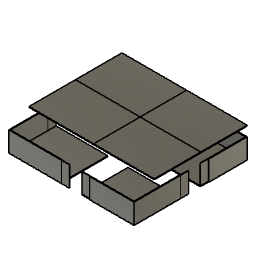
cajav3 v2 (Autodesk Fusion 360 design; units mm, degrees)
Autodesk Fusion 360 part; units mm, degrees
note: some values were not read from the file. Chosen so that the rebuilt part matches the saved one: which bodies a step acts on; which face or edge a step refers to.
sketch "Boceto1" plane through (0, 0, 0) normal (0, 0, 1) x (1, 0, 0)
  line L0 (0, 0) -> (-260, 0)
  line L1 (-260, 0) -> (-260, 230)
  line L2 (-260, 230) -> (0, 230)
  line L3 (0, 230) -> (0, 0)
  dimension "d1" = 230
  constraint horizontal L0
  constraint vertical L1
  constraint horizontal L2
  constraint vertical L3
  constraint coincident L0.start L3.end
  measures "d1" distance of L0.start L2.end
extrude "Extruir1" add sketch "Boceto1" along normal blind 50 and the other way blind 0 makes body 1
shell "Vaciado1" thickness 2 removed faces 1 at (-86.6667, 76.6667, 50) on bodies 1
ref_plane "PlanoDeObra1" through (-130, 0, 0) normal (1, 0, 0) x (0, 1, 0)
split "Dividir1" by plane through (-130, 0, 0) normal (1, 0, 0) bodies 1 makes body 2 at (-43.3333, 153.3333, 0)
move_body "Desplazar1" bodies 2 to x (1, 0, 0) y (0, 1, 0) z (0, 0, 1) at (50, 0, 0)
sketch "Boceto2" plane through (0, 0, 50) normal (0, 0, 1) x (-1, 0, 0)
  line L0 (80, -2) -> (80, 0)
  line L1 (80, 0) -> (-50, 0)
  line L2 (-50, 0) -> (-50, -230)
  line L3 (-50, -230) -> (80, -230)
  line L4 (80, -230) -> (80, -228)
  line L5 (80, -228) -> (-48, -228)
  line L6 (-48, -228) -> (-48, -2)
  line L7 (-48, -2) -> (80, -2)
  line L8 (80, 0) -> (60, 0)
  line L9 (60, 0) -> (60, -1)
  line L10 (60, -1) -> (80, -1)
  line L11 (80, -1) -> (80, 0)
  constraint horizontal L8
  constraint vertical L9
  constraint horizontal L10
  constraint vertical L11
  constraint coincident L0.end L1.start
extrude "Extruir2" cut sketch "Boceto2" against normal blind 51 contours L0 L1 L8 L9 L10 L11 bodies 2
sketch "Boceto3" plane through (-130, 0, 0) normal (1, 0, 0) x (0, 1, 0)
  line L0 (230, 0) -> (230, 50)
  line L1 (230, 50) -> (228, 50)
  line L2 (228, 50) -> (228, 2)
  line L3 (228, 2) -> (2, 2)
  line L4 (2, 2) -> (2, 50)
  line L5 (2, 50) -> (0, 50)
  line L6 (0, 50) -> (0, 0)
  line L7 (0, 0) -> (230, 0)
  line L8 (0, 0) -> (1, 0)
  line L9 (1, 0) -> (1, 50)
  line L10 (1, 50) -> (0, 50)
  line L11 (0, 50) -> (0, 0)
  dimension "d10" = 1
  constraint horizontal L8
  constraint vertical L9
  constraint horizontal L10
  constraint vertical L11
  constraint coincident L5 L9.end
  constraint coincident L6.end L7.start
  measures "d10" distance of L6.end L8.end
extrude "Extruir3" add sketch "Boceto3" along normal blind 20 and the other way blind 0 contours L5 L6 L7 L8 L9 L10 L11 bodies 1
sketch "Boceto4" plane through (-80, 0, 0) normal (-1, 0, 0) x (0, -1, 0)
  line L0 (-1, 0) -> (-1, 50)
  line L1 (-1, 50) -> (-2, 50)
  line L2 (-2, 50) -> (-2, 2)
  line L3 (-2, 2) -> (-228, 2)
  line L4 (-228, 2) -> (-228, 50)
  line L5 (-228, 50) -> (-230, 50)
  line L6 (-230, 50) -> (-230, 0)
  line L7 (-230, 0) -> (-1, 0)
  line L8 (-230, 0) -> (-229, 0)
  line L9 (-229, 0) -> (-229, 50)
  line L10 (-229, 50) -> (-230, 50)
  line L11 (-230, 50) -> (-230, 0)
  dimension "d15" = 1
  constraint horizontal L8
  constraint vertical L9
  constraint horizontal L10
  constraint vertical L11
  constraint coincident L5 L9.end
  constraint coincident L6.end L7.start
  measures "d15" distance of L6.end L8.end
extrude "Extruir4" cut sketch "Boceto4" along normal blind 0 and the other way blind 20 contours L5 L6 L7 L8 L9 L10 L11 bodies 2
sketch "Boceto5" plane through (-130, 0, 0) normal (1, 0, 0) x (0, 1, 0)
  line L0 (1, 50) -> (1, 0)
  line L1 (1, 0) -> (230, 0)
  line L2 (230, 0) -> (230, 50)
  line L3 (230, 50) -> (228, 50)
  line L4 (228, 50) -> (228, 2)
  line L5 (228, 2) -> (2, 2)
  line L6 (2, 2) -> (2, 50)
  line L7 (2, 50) -> (1, 50)
  line L8 (230, 0) -> (229, 0)
  line L9 (229, 0) -> (229, 50)
  line L10 (229, 50) -> (230, 50)
  line L11 (230, 50) -> (230, 0)
  dimension "d20" = 1
  constraint horizontal L8
  constraint vertical L9
  constraint horizontal L10
  constraint vertical L11
  constraint coincident L3 L9.end
  constraint coincident L1.end L2.start
  measures "d20" distance of L1.end L8.end
extrude "Extruir5" add sketch "Boceto5" along normal blind 20 and the other way blind 0 contours L1 L2 L3 L8 L9 L10 L11 bodies 1
sketch "Boceto8" plane through (0, 0, 0) normal (0, 0, 1) x (1, 0, 0)
  line L0 (50, 0) -> (-260, 0)
  line L1 (-260, 0) -> (-260, 230)
  line L2 (-260, 230) -> (50, 230)
  line L3 (50, 230) -> (50, 0)
  constraint horizontal L0
  constraint vertical L1
  constraint horizontal L2
  constraint vertical L3
extrude "Extruir8" add sketch "Boceto8" along normal blind 73 and the other way blind -75 separate body makes body 3
ref_plane "PlanoDeObra2" through (0, 115, 0) normal (0, 1, 0) x (0, 0, 1)
ref_plane "PlanoDeObra3" through (-100, 0, 0) normal (1, 0, 0) x (0, 1, 0)
split "Dividir2" by plane through (-100, 0, 0) normal (1, 0, 0) bodies 3 makes body 4 at (0, 76.6667, 75)
split "Dividir3" by plane through (0, 115, 0) normal (0, 1, 0) bodies 2 4 1 3 makes body 7 at (-153.3333, 153.3333, 75) makes body 5 at (-216.6667, 191.3333, 0) makes body 8 at (-50, 153.3333, 75) makes body 6 at (-30, 153, 0)
move_body "Desplazar2" bodies 2 to x (1, 0, 0) y (0, 1, 0) z (0, 0, 1) at (0, -50, 0)
move_body "Desplazar3" bodies 1 to x (1, 0, 0) y (0, 1, 0) z (0, 0, 1) at (0, -50, 0)
sketch "Boceto9" plane through (0, 115, 0) normal (0, -1, 0) x (1, 0, 0)
  line L0 (-258, 50) -> (-260, 50)
  line L1 (-260, 50) -> (-260, 0)
  line L2 (-260, 0) -> (-130, 0)
  line L3 (-130, 0) -> (-130, 2)
  line L4 (-130, 2) -> (-258, 2)
  line L5 (-258, 2) -> (-258, 50)
  line L6 (-260, 0) -> (-259, 0)
  line L7 (-259, 0) -> (-259, 50)
  line L8 (-259, 50) -> (-260, 50)
  line L9 (-260, 50) -> (-260, 0)
  dimension "d40" = 1
  constraint horizontal L6
  constraint vertical L7
  constraint horizontal L8
  constraint vertical L9
  constraint coincident L0 L7.end
  constraint coincident L1.end L2.start
  measures "d40" distance of L1.end L6.end
extrude "Extruir9" add sketch "Boceto9" along normal blind 20 and the other way blind 0 contours L0 L1 L2 L6 L7 L8 L9 bodies 5
sketch "Boceto10" plane through (0, 65, 0) normal (0, 1, 0) x (-1, 0, 0)
  line L0 (260, 50) -> (258, 50)
  line L1 (258, 50) -> (258, 2)
  line L2 (258, 2) -> (130, 2)
  line L3 (130, 2) -> (130, 0)
  line L4 (130, 0) -> (260, 0)
  line L5 (260, 0) -> (260, 50)
  line L6 (260, 0) -> (259, 0)
  line L7 (259, 0) -> (259, 50)
  line L8 (259, 50) -> (260, 50)
  line L9 (260, 50) -> (260, 0)
  dimension "d45" = 1
  constraint horizontal L6
  constraint vertical L7
  constraint horizontal L8
  constraint vertical L9
  constraint coincident L0 L7.end
  constraint coincident L4.end L5.start
  measures "d45" distance of L4.end L6.end
extrude "Extruir10" cut sketch "Boceto10" along normal blind 0 and the other way blind 20 contours L0 L4 L5 L6 L7 L8 L9 bodies 1
sketch "Boceto11" plane through (0, 65, 0) normal (0, 1, 0) x (-1, 0, 0)
  line L0 (80, 0) -> (80, 2)
  line L1 (80, 2) -> (-48, 2)
  line L2 (-48, 2) -> (-48, 50)
  line L3 (-48, 50) -> (-50, 50)
  line L4 (-50, 50) -> (-50, 0)
  line L5 (-50, 0) -> (80, 0)
  line L6 (-50, 0) -> (-49, 0)
  line L7 (-49, 0) -> (-49, 50)
  line L8 (-49, 50) -> (-50, 50)
  line L9 (-50, 50) -> (-50, 0)
  dimension "d50" = 1
  constraint horizontal L6
  constraint vertical L7
  constraint horizontal L8
  constraint vertical L9
  constraint coincident L3 L7.end
  constraint coincident L4.end L5.start
  measures "d50" distance of L4.end L6.end
extrude "Extruir11" add sketch "Boceto11" along normal blind 20 and the other way blind 0 contours L3 L4 L5 L6 L7 L8 L9 bodies 2
sketch "Boceto12" plane through (0, 115, 0) normal (0, 1, 0) x (1, 0, 0)
  line L0 (50, 0) -> (49, 0)
  line L1 (49, 0) -> (49, -50.1802)
  line L2 (49, -50.1802) -> (50, -50.1802)
  line L3 (50, -50.1802) -> (50, 0)
  dimension "d55" = 1
  constraint horizontal L0
  constraint vertical L1
  constraint horizontal L2
  constraint vertical L3
  measures "d55" distance of L0.start L0.end
extrude "Extruir12" cut sketch "Boceto12" along normal blind 20 and the other way blind 5 bodies 6
